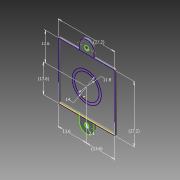
# Autodesk Inventor part: CameraLensHolder
Saved by Autodesk Inventor 2015 (Build 190159000, 159)
## iProperties
Created: 2015-03-20
Part Number: CameraLensHolder
Material: Generic
Document SubType Name: Modeling
Designer: Akovo_000
Density: 1 g/cm^3
Appearance: Default
Author: Akovo_000
Autodesk Inventor part; units mm, degrees
ref_plane "YZ Plane" through (0, 0, 0) normal (1, 0, 0) x (0, 1, 0)
ref_plane "XZ Plane" through (0, 0, 0) normal (0, 1, 0) x (-1, 0, 0)
ref_plane "XY Plane" through (0, 0, 0) normal (0, 0, 1) x (1, 0, 0)
sketch "Sketch1" plane through (0, 0, 0) normal (0, 1, 0) x (-1, 0, 0)
  line L0 (12.0321, 17.9508) -> (-14.4679, 17.9508)
  line L1 (-14.4679, 17.9508) -> (-14.4679, -8.5492)
  line L2 (-14.4679, -8.5492) -> (12.0321, -8.5492)
  line L3 (12.0321, -8.5492) -> (12.0321, 17.9508)
  line L4 (12.3821, 18.3008) -> (-14.8179, 18.3008)
  line L5 (-14.8179, 18.3008) -> (-14.8179, -8.8992)
  line L6 (-14.8179, -8.8992) -> (12.3821, -8.8992)
  line L7 (12.3821, -8.8992) -> (12.3821, 18.3008)
  line L8 (12.0321, -8.5492) -> (-14.4679, -8.5492)
  line L9 (12.3821, -8.8992) -> (-14.8179, -8.8992)
  line L10 (-1.2179, 18.3008) -> (2.2821, 18.3008)
  line L11 (2.2821, 18.3008) -> (2.2821, 20.8008)
  line L12 (-1.2179, 18.3008) -> (-4.7179, 18.3008)
  line L13 (-4.7179, 18.3008) -> (-4.7179, 20.8008)
  arc A0 (2.2821, 20.8008) -> (-4.7179, 20.8008) centre (-1.2179, 20.8008) ccw
  line L14 (-1.2179, -8.8992) -> (-4.7179, -8.8992)
  line L15 (-4.7179, -8.8992) -> (-4.7179, -11.3992)
  line L16 (-1.2179, -8.8992) -> (2.2821, -8.8992)
  line L17 (2.2821, -8.8992) -> (2.2821, -11.3992)
  arc A1 (-4.7179, -11.3992) -> (2.2821, -11.3992) centre (-1.2179, -11.3992) ccw
  circle A2 centre (-1.2179, 20.8008) radius 1.05
  circle A3 centre (-1.2179, -11.3992) radius 1.05
  point P0 (0, 0)
  point P1 (12.0321, 4.7008)
  point P2 (-14.4679, 4.7008)
  dimension "d0" = 26.5
  dimension "d1" = 26.5
  dimension "d2" = 27.2
  dimension "d3" = 27.2
  dimension "d4" = 0.35
  dimension "d5" = 0.35
  dimension "d6" = 0.35
  dimension "d7" = 0.35
  dimension "d39" = 2.5
  dimension "d41" = 3.5
  dimension "d43" = 2.5
  dimension "d45" = 3.5
  dimension "d46" = 2.1
  dimension "d53" = 2.1
  constraints: 36 end point, 6 horizontal, 6 perpendicular, 4 centre point, 4 midpoint, 4 parallel, 4 point on circle, 2 coincident
  measures "d0" distance of L2.end L1.end
  measures "d1" distance of L1.end L0.end
  measures "d2" distance of L6.end L5.end
  measures "d3" distance of L5.end L4.end
  measures "d4" distance between parallel lines of L4 L0
  measures "d5" distance between parallel lines of L3 L7
  measures "d6" distance between parallel lines of L5 L1
  measures "d7" distance between parallel lines of L2 L6
  measures "d39" distance of L11.end L10.end
  measures "d41" radius of A0
  measures "d43" distance of L15.end L14.end
  measures "d45" radius of A1
  measures "d46" diameter of A2
  measures "d53" diameter of A3
extrude "Director" add sketch "Sketch1" along normal blind 1
sketch "Sketch3" plane through (0, 0, 0) normal (0, -1, 0) x (1, 0, 0)
  line L0 (-12.3821, 18.3008) -> (14.8179, 18.3008)
  line L1 (14.8179, 18.3008) -> (14.8179, -8.8992)
  line L2 (14.8179, -8.8992) -> (-12.3821, -8.8992)
  line L3 (-12.3821, -8.8992) -> (-12.3821, 18.3008)
  line L4 (-2.2821, 18.3008) -> (-2.2821, 20.8008)
  line L5 (4.7179, 18.3008) -> (4.7179, 20.8008)
  arc A0 (4.7179, 20.8008) -> (-2.2821, 20.8008) centre (1.2179, 20.8008) ccw
  line L6 (-2.2821, -11.3992) -> (-2.2821, -8.8992)
  line L7 (4.7179, -8.8992) -> (4.7179, -11.3992)
  arc A1 (-2.2821, -11.3992) -> (4.7179, -11.3992) centre (1.2179, -11.3992) ccw
  circle A2 centre (1.2179, -11.3992) radius 1.05
  circle A3 centre (1.2179, 20.8008) radius 1.05
  line L8 (-12.3821, -8.8992) -> (-12.3821, 18.3008) projected
  line L9 (14.8179, 18.3008) -> (14.8179, -8.8992) projected
  circle A4 centre (1.2179, 4.7008) radius 7
  circle A5 centre (1.2179, 4.7008) radius 5.9
  line L10 (-2.2821, 18.3008) -> (4.7179, 18.3008)
  line L11 (4.7179, -8.8992) -> (-2.2821, -8.8992)
  line L12 (-12.0321, -8.5492) -> (14.4679, -8.5492) projected
  point P0 (0, 0)
  dimension "d59" = 2.1
  dimension "d61" = 14
  dimension "d62" = 11.8
  dimension "d63" = 13.6
  dimension "d64" = 13.6
  dimension "d65" = 27.2
  dimension "d66" = 27.2
  dimension "d67" = 13.6
  dimension "d68" = 13.6
  constraints: 20 end point, 6 centre point, 4 point on circle, 4 tangent, 3 coincident, 3 parallel, 1 collinear, 1 horizontal, 1 perpendicular
  measures "d59" diameter of A2
  measures "d61" diameter of A4
  measures "d62" diameter of A5
  measures "d63" distance from line of L3 A4.centre
  measures "d64" distance from line of A5.centre L1
  measures "d65" distance between parallel lines of L1 L3
  measures "d66" distance between parallel lines of L2 L0
  measures "d67" distance from line of L0 A4.centre
  measures "d68" distance from line of L2 A4.centre
body "Solid4"
